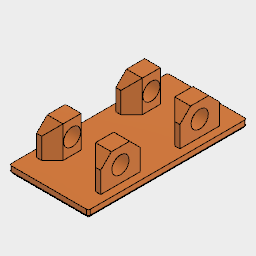
prusa_i3_bear_upgrade (Autodesk Fusion 360 archive; units mm, degrees)
design "end_cap"
Autodesk Fusion 360 part; units mm, degrees
sketch "base" plane through (0, 0, 0) normal (0, 0, 1) x (1, 0, 0)
  line L0 (0, 0) -> (20, 0)
  line L1 (20, 0) -> (20, 40)
  line L2 (20, 40) -> (0, 40)
  line L3 (0, 40) -> (0, 0)
  line L4 (10, 0) -> (10, 40) construction
  line L5 (1.9, 15) -> (5.9, 15)
  line L6 (5.9, 15) -> (5.9, 5)
  line L7 (5.9, 5) -> (1.9, 5)
  line L8 (1.9, 5) -> (1.9, 15)
  line L9 (14.1, 15) -> (18.1, 15)
  line L10 (18.1, 15) -> (18.1, 5)
  line L11 (18.1, 5) -> (14.1, 5)
  line L12 (14.1, 5) -> (14.1, 15)
  line L13 (0, 10) -> (20, 10) construction
  line L14 (0, 20) -> (20, 20) construction
  line L15 (5.9, 25) -> (5.9, 35)
  line L16 (5.9, 35) -> (1.9, 35)
  line L17 (1.9, 25) -> (5.9, 25)
  line L18 (1.9, 35) -> (1.9, 25)
  line L19 (18.1, 25) -> (18.1, 35)
  line L20 (18.1, 35) -> (14.1, 35)
  line L21 (14.1, 25) -> (18.1, 25)
  line L22 (14.1, 35) -> (14.1, 25)
  dimension "d2505" = 20
  dimension "d2506" = 40
  dimension "d2525" = 0
  dimension "d2526" = 0
  dimension "d2527" = 0
  dimension "d2528" = 0
  dimension "d2539" = 0
  dimension "d2540" = 0
  dimension "d2541" = 0
  dimension "d2542" = 0
  dimension "d2551" = 0
  dimension "d2552" = 0
  dimension "d2553" = 0
  dimension "d2554" = 0
  dimension "d2563" = 0
  dimension "d2564" = 0
  dimension "d2565" = 0
  dimension "d2566" = 0
  dimension "d2" = 10
  dimension "d3" = 4
  dimension "d4" = 10
  dimension "d5" = 4
  dimension "d6" = 10
  dimension "d7" = 1.9
  dimension "d8" = 1.9
  dimension "d12" = 20
  measures "d2505" distance of L0.start L0.end
  measures "d2506" distance of L0.start L2.end
  measures "d2" distance of L5.end L6.end
  measures "d3" distance of L5.start L5.end
  measures "d4" distance of L9.start L11.end
  measures "d5" distance of L9.start L9.end
  measures "d6" distance of L0 L13
  measures "d7" distance of L3 L8
  measures "d8" distance of L1 L10
  measures "d12" distance of L2 L14
extrude "Extrude1" add sketch "base" along normal blind 2 contours L0 L1 L2 L3 | L5 L6 L7 L8 | L9 L10 L11 L12 | L15 L16 L17 L18 | L19 L20 L21 L22
extrude "Extrude2" add sketch "base" along normal up to surface (10 mm away) contours L5 L6 L7 L8 | L9 L10 L11 L12 | L15 L16 L17 L18 | L19 L20 L21 L22
sketch "holes" plane through (0, 0, 0) normal (-1, 0, 0) x (0, -1, 0)
  line L0 (0, 2) -> (-40, 2)
  line L1 (-15, 2) -> (-15, 10)
  line L2 (-15, 2) -> (-5, 2)
  line L3 (-5, 2) -> (-5, 10)
  line L4 (-5, 10) -> (-15, 10)
  line L5 (-15, 10) -> (-15, 2)
  line L6 (-15, 6) -> (-5, 6) construction
  circle A0 centre (-10, 6) radius 2.175
  line L7 (-40, 0) -> (0, 0)
  line L8 (0, 0) -> (0, 2)
  line L9 (-40, 2) -> (-40, 0)
  line L10 (-35, 2) -> (-25, 2)
  line L11 (-25, 2) -> (-25, 10)
  line L12 (-25, 10) -> (-35, 10)
  line L13 (-35, 10) -> (-35, 2)
  line L14 (-35, 6) -> (-25, 6) construction
  circle A1 centre (-30, 6) radius 2.175
  dimension "d9" = 4.35
  dimension "d13" = 4.35
  measures "d9" diameter of A0
  measures "d13" diameter of A1
extrude "Extrude5" cut sketch "holes" against normal up to surface (20 mm away) contours A0 | A1
fillet "Fillet1" radius 0.5 4 edges at (20, 40, 1) (0, 40, 1) (0, 0, 1) (20, 0, 1)
chamfer "Chamfer1" distance 2.7 angle 45 16 edges at (5.9, 5, 6) (3.9, 5, 10) (3.9, 15, 10) (5.9, 15, 6) (16.1, 15, 10) (16.1, 5, 10) (14.1, 5, 6) (14.1, 15, 6) (5.9, 25, 6) (14.1, 25, 6) (3.9, 25, 10) (16.1, 25, 10) (16.1, 35, 10) (14.1, 35, 6) (5.9, 35, 6) (3.9, 35, 10)
sketch "bear" plane through (0, 0, 0) normal (0, 0, -1) x (1, 0, 0)
  arc A0 (20, -0.5) -> (19.5, 0) centre (19.5, -0.5) ccw
  line L0 (19.5, 0) -> (0.5, 0)
  arc A1 (0.5, 0) -> (0, -0.5) centre (0.5, -0.5) ccw
  line L1 (0, -0.5) -> (0, -39.5)
  arc A2 (0, -39.5) -> (0.5, -40) centre (0.5, -39.5) ccw
  line L2 (0.5, -40) -> (19.5, -40)
  arc A3 (19.5, -40) -> (20, -39.5) centre (19.5, -39.5) ccw
  line L3 (20, -39.5) -> (20, -0.5)
  spline S0 degree 5 poles (9.966, -9.8106) (10.0307, -9.8106) (10.1684, -9.8018) (10.4002, -9.7624) (10.7537, -9.6582) (11.2372, -9.4515) (11.7261, -9.1858) (12.1914, -8.8873) (12.6273, -8.5936) (13.0463, -8.3489) (13.4677, -8.1963) (13.9085, -8.1718) (14.3719, -8.2972) (14.8428, -8.5761) (15.2947, -8.999) (15.695, -9.5463) (16.0101, -10.1916) (16.2113, -10.9054) (16.2794, -11.6578) (16.209, -12.4202) (16.0114, -13.168) (15.7222, -13.8822) (15.3966, -14.5517) (15.1369, -15.1757) (15.0089, -15.7636) (15.0284, -16.33) (15.1825, -16.8916) (15.4362, -17.4636) (15.7454, -18.0556) (16.0669, -18.6687) (16.3609, -19.2975) (16.5931, -19.9328) (16.7373, -20.5637) (16.7772, -21.1803) (16.7099, -21.7758) (16.546, -22.3484) (16.3066, -22.8993) (16.0201, -23.4315) (15.7195, -23.9484) (15.4391, -24.4521) (15.2113, -24.9429) (15.0636, -25.4207) (15.0135, -25.887) (15.066, -26.3466) (15.2079, -26.8103) (15.4098, -27.293) (15.6325, -27.8087) (15.8324, -28.3659) (15.9677, -28.9632) (16.0042, -29.5842) (15.9174, -30.2003) (15.6941, -30.777) (15.3335, -31.2788) (14.8486, -31.674) (14.2686, -31.9409) (13.634, -32.0695) (12.9888, -32.0625) (12.3726, -31.9358) (11.8135, -31.7192) (11.319, -31.4585) (10.8754, -31.2111) (10.5431, -31.0686) (10.2967, -31.0125) (10.1323, -31) (10.05, -31) knots 0 0 0 0 0 0 0.01666667 0.03333333 0.05 0.06666667 0.08333333 0.1 0.11666667 0.13333333 0.15 0.16666667 0.18333333 0.2 0.21666667 0.23333333 0.25 0.26666667 0.28333333 0.3 0.31666667 0.33333333 0.35 0.36666667 0.38333333 0.4 0.41666667 0.43333333 0.45 0.46666667 0.48333333 0.5 0.51666667 0.53333333 0.55 0.56666667 0.58333333 0.6 0.61666667 0.63333333 0.65 0.66666667 0.68333333 0.7 0.71666667 0.73333333 0.75 0.76666667 0.78333333 0.8 0.81666667 0.83333333 0.85 0.86666667 0.88333333 0.9 0.91666667 0.93333333 0.95 0.96666667 0.98333333 1 1 1 1 1 1
  line L4 (8.166, -9.8106) -> (11.766, -9.8106)
  line L5 (16.65, -11.8) -> (14.3026, -16.9967)
  line L6 (12.25, -31) -> (7.85, -31)
  line L7 (9.966, -9.8106) -> (10.05, -31) construction
  spline S1 degree 5 poles (9.966, -9.8106) (9.9013, -9.8111) (9.7635, -9.8034) (9.5314, -9.7658) (9.1772, -9.6645) (8.692, -9.4616) (8.2011, -9.1997) (7.7334, -8.9049) (7.2952, -8.6148) (6.8742, -8.3734) (6.4517, -8.2241) (6.0107, -8.2032) (5.5482, -8.3322) (5.0796, -8.6148) (4.631, -9.0413) (4.2351, -9.5917) (3.9251, -10.2395) (3.7296, -10.9549) (3.6674, -11.7078) (3.7439, -12.4696) (3.9475, -13.2158) (4.2422, -13.9277) (4.5732, -14.5946) (4.8378, -15.2165) (4.9705, -15.8034) (4.9555, -16.3699) (4.8058, -16.9328) (4.5567, -17.5067) (4.2522, -18.1012) (3.9355, -18.7168) (3.6465, -19.3479) (3.4193, -19.985) (3.2802, -20.617) (3.2451, -21.2339) (3.3172, -21.8288) (3.4856, -22.4002) (3.7294, -22.9492) (4.0201, -23.4791) (4.3248, -23.9935) (4.6092, -24.4951) (4.8408, -24.984) (4.9923, -25.4606) (5.0461, -25.9265) (4.9973, -26.3865) (4.859, -26.8513) (4.661, -27.3356) (4.4424, -27.8531) (4.2469, -28.4118) (4.1163, -29.0102) (4.0848, -29.6314) (4.1764, -30.2468) (4.4043, -30.8218) (4.7689, -31.3207) (5.2569, -31.712) (5.839, -31.9743) (6.4746, -32.0979) (7.1197, -32.0858) (7.7349, -31.9542) (8.2923, -31.7332) (8.7847, -31.4685) (9.2263, -31.2176) (9.5575, -31.0725) (9.8034, -31.0144) (9.9677, -31.0007) (10.05, -31) knots 0 0 0 0 0 0 0.01666667 0.03333333 0.05 0.06666667 0.08333333 0.1 0.11666667 0.13333333 0.15 0.16666667 0.18333333 0.2 0.21666667 0.23333333 0.25 0.26666667 0.28333333 0.3 0.31666667 0.33333333 0.35 0.36666667 0.38333333 0.4 0.41666667 0.43333333 0.45 0.46666667 0.48333333 0.5 0.51666667 0.53333333 0.55 0.56666667 0.58333333 0.6 0.61666667 0.63333333 0.65 0.66666667 0.68333333 0.7 0.71666667 0.73333333 0.75 0.76666667 0.78333333 0.8 0.81666667 0.83333333 0.85 0.86666667 0.88333333 0.9 0.91666667 0.93333333 0.95 0.96666667 0.98333333 1 1 1 1 1 1
  line L8 (11.766, -9.7963) -> (8.1661, -9.8249)
  line L9 (3.298, -11.8529) -> (5.6865, -17.0308)
  line L10 (7.8501, -31.0174) -> (12.2499, -30.9826)
  circle A4 centre (12.5483, -27.3765) radius 0.7448
  ellipse E0 centre (10.0265, -25.0801) end of major axis (8.2046, -25.0873) minor radius 1.3284
  line L11 (11.8485, -25.0728) -> (8.2046, -25.0873)
  line L12 (10.0213, -23.7517) -> (10.0318, -26.4085)
  circle A5 centre (7.523, -27.3965) radius 0.7448
  ellipse E1 centre (14.4043, -20.6952) end of major axis (14.4043, -18.6032) minor radius 1.5739
  line L13 (14.4043, -22.7872) -> (14.4043, -18.6032)
  line L14 (15.9782, -20.6952) -> (12.8304, -20.6952)
  ellipse E2 centre (5.6142, -20.73) end of major axis (5.5976, -18.6381) minor radius 1.5739
  ellipse E3 centre (13.9043, -11.1952) end of major axis (13.9043, -9.1032) minor radius 1.5739
  ellipse E4 centre (6.0388, -11.2264) end of major axis (6.0223, -9.1344) minor radius 1.5739
  point P0 (13.75, -8.2)
  point P1 (15.85, -9.9)
  point P2 (15.4763, -14.3983)
  point P3 (15.4416, -17.4507)
  point P4 (16.75, -21)
  point P5 (15.75, -23.9)
  point P6 (15.05, -26.1)
  point P7 (15.85, -28.5)
  point P8 (15.15, -31.4)
  point P9 (12.05, -31.8)
  point P10 (11.85, -9.1)
  point P11 (8.0764, -9.115)
  point P12 (6.1694, -8.23)
  point P13 (4.0829, -9.9466)
  point P14 (4.4923, -14.4419)
  point P15 (4.5511, -17.4939)
  point P16 (3.2709, -21.0534)
  point P17 (4.2939, -23.9454)
  point P18 (5.0113, -26.1398)
  point P19 (4.2304, -28.5461)
  point P20 (4.9533, -31.4404)
  point P21 (8.0564, -31.8158)
extrude "Extrude4" cut sketch "bear" against normal blind 1 contours S0 S1
chamfer "Chamfer2" distance 0.7 angle 35 8 edges at (10, 40, 0) (0.1464, 39.8536, 0) (0, 20, 0) (0.1464, 0.1464, 0) (10, 0, 0) (19.8536, 0.1464, 0) (20, 20, 0) (19.8536, 39.8536, 0) measured on face at (13.1667, 40, 1.3333) measured on face at (0.0141, 39.6179, 0.6667) measured on face at (0, 26.5, 1.3333) measured on face at (0.4762, 0.0006, 0.6667) measured on face at (6.8333, 0, 0.6667) measured on face at (19.8619, 0.155, 0.6667) measured on face at (20, 13.5, 1.3333) measured on face at (19.991, 39.5946, 0.6667)
equation "d4 = d2"
equation "d5 = d3"
equation "d8 = d7"
equation "d13 = d9"

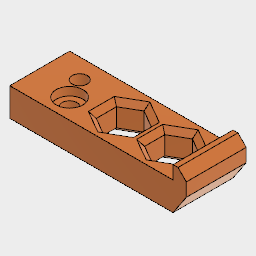
design "psu_upper_mount"
Autodesk Fusion 360 part; units mm, degrees
sketch "base" plane through (0, 0, 0) normal (0, 0, 1) x (1, 0, 0)
  circle A0 centre (9, 12.025) radius 2.25
  circle A1 centre (12, 5.975) radius 2.25
  circle A2 centre (12, 5.975) radius 4
  circle A3 centre (9, 12.025) radius 3.6 construction
  line L0 (5.8823, 10.225) -> (9, 8.425)
  line L1 (9, 8.425) -> (12.1177, 10.225)
  line L2 (12.1177, 10.225) -> (12.1177, 13.825)
  line L3 (12.1177, 13.825) -> (9, 15.625)
  line L4 (9, 15.625) -> (5.8823, 13.825)
  line L5 (5.8823, 13.825) -> (5.8823, 10.225)
  line L6 (0, 18) -> (53, 18)
  line L7 (53, 18) -> (53, 0)
  line L8 (53, 0) -> (0, 0)
  line L9 (0, 0) -> (0, 18)
  line L10 (49, 18) -> (49, 0)
  line L11 (0, 9) -> (49, 9) construction
  point P0 (9, 12.025)
  dimension "d1" = 4.5
  dimension "d2" = 4.5
  dimension "d3" = 8
  dimension "d6" = 7.2
  dimension "d8" = 4
  dimension "d9" = 18
  dimension "d22" = 49
  dimension "d23" = 40
  dimension "d31" = 6.05
  dimension "d33" = 3
  dimension "d34" = 3.025
  measures "d1" diameter of A0
  measures "d2" diameter of A1
  measures "d3" diameter of A2
  measures "d6" diameter of A3
  measures "d8" distance of L7 L10
  measures "d9" distance of L6.start L8.end
  measures "d22" distance of L9 L10
  measures "d23" distance of P0 L10
  measures "d31" distance of P0 A1.centre
  measures "d33" distance of P0 A1.centre
  measures "d34" distance of P0 L11.start
extrude "Extrude1" add sketch "base" along normal blind 8.5 contours A2 L0 L1 | A2 L0 L1 | A2 L0 L1 L2 L3 L4 L5 | L6 L8 L9 L10
extrude "Extrude2" add sketch "base" along normal up to surface (12.5 mm away) contours L6 L7 L8 L10
extrude "Extrude3" cut sketch "base" along normal blind 4 contours A2 L0 L1 | A2 L0 L1 L2 L3 L4 L5 picked at (10.5961, 9.4215)
extrude "Extrude4" cut sketch "base" against normal blind 2.5 from surface at 8.5 contours A2 L0 L1 | A2 L0 L1
sketch "poly" plane through (0, 0, 8.5) normal (0, 0, 1) x (-1, 0, 0)
  circle A0 centre (-12, -5.975) radius 4
  circle A1 centre (-9, -12.025) radius 2.25
  line L0 (-49, -18) -> (0, -18)
  line L1 (0, -18) -> (0, 0)
  line L2 (0, 0) -> (-49, 0)
  line L3 (-49, 0) -> (-49, -18)
  line L4 (-49, -18) -> (-49, 0)
  line L5 (-49, -9) -> (-16, -9) construction
  line L6 (-49, -18) -> (0, -18)
  line L7 (0, 0) -> (-49, 0)
  line L8 (-16, -18) -> (-16, 0) construction
  line L9 (-25.25, -15.0622) -> (-20, -12.0311)
  line L10 (-20, -12.0311) -> (-20, -5.9689)
  line L11 (-20, -5.9689) -> (-25.25, -2.9378)
  line L12 (-25.25, -2.9378) -> (-30.5, -5.9689)
  line L13 (-30.5, -5.9689) -> (-30.5, -12.0311)
  line L14 (-30.5, -12.0311) -> (-25.25, -15.0622)
  line L15 (-34.5, -12.0311) -> (-34.5, -5.9689)
  line L16 (-34.5, -5.9689) -> (-39.75, -2.9378)
  line L17 (-39.75, -2.9378) -> (-45, -5.9689)
  line L18 (-45, -5.9689) -> (-45, -12.0311)
  line L19 (-45, -12.0311) -> (-39.75, -15.0622)
  line L20 (-39.75, -15.0622) -> (-34.5, -12.0311)
  line L21 (-39.75, -9) -> (-42.375, -13.5466) construction
  circle A2 centre (-12, -5.975) radius 4
  point P0 (-25.25, -9)
  point P1 (-39.75, -9)
  dimension "d25" = 4
  dimension "d26" = 4
  dimension "d27" = 4
  measures "d25" distance of L8 L10
  measures "d26" distance of L3 L18
  measures "d27" distance of L13 L15
extrude "Extrude5" cut sketch "poly" against normal up to surface (8.5 mm away) contours L9 L10 L11 L12 L13 L14 | L15 L16 L17 L18 L19 L20
chamfer "Chamfer1" distance 2.5 angle 45 1 edges at (53, 9, 12.5)
chamfer "Chamfer2" distance 1.5 angle 45 24 edges at (27.875, 4.4534, 8.5) (30.5, 9, 8.5) (27.875, 13.5466, 8.5) (22.625, 13.5466, 8.5) (20, 9, 8.5) (22.625, 4.4534, 8.5) (22.625, 4.4534, 0) (27.875, 4.4534, 0) (30.5, 9, 0) (34.5, 9, 8.5) (37.125, 4.4534, 0) (37.125, 4.4534, 8.5) (42.375, 4.4534, 0) (42.375, 4.4534, 8.5) (45, 9, 0) (45, 9, 8.5) (42.375, 13.5466, 8.5) (37.125, 13.5466, 8.5) (27.875, 13.5466, 0) (22.625, 13.5466, 0) (20, 9, 0) (37.125, 13.5466, 0) (34.5, 9, 0) (42.375, 13.5466, 0) measured on face at (2.2833, 9.7873, 8.5) measured on face at (2.2833, 9.7873, 8.5) measured on face at (2.2833, 9.7873, 8.5) measured on face at (2.2833, 9.7873, 8.5) measured on face at (2.2833, 9.7873, 8.5) measured on face at (2.2833, 9.7873, 8.5) measured on face at (50.3333, 10.0104, 0) measured on face at (50.3333, 10.0104, 0) measured on face at (50.3333, 10.0104, 0) measured on face at (2.2833, 9.7873, 8.5) measured on face at (50.3333, 10.0104, 0) measured on face at (2.2833, 9.7873, 8.5) measured on face at (50.3333, 10.0104, 0) measured on face at (2.2833, 9.7873, 8.5) measured on face at (50.3333, 10.0104, 0) measured on face at (2.2833, 9.7873, 8.5) measured on face at (2.2833, 9.7873, 8.5) measured on face at (2.2833, 9.7873, 8.5) measured on face at (50.3333, 10.0104, 0) measured on face at (50.3333, 10.0104, 0) measured on face at (50.3333, 10.0104, 0) measured on face at (50.3333, 10.0104, 0) measured on face at (50.3333, 10.0104, 0) measured on face at (50.3333, 10.0104, 0)
chamfer "Chamfer3" distance 4 distance2 6 1 edges at (53, 9, 0) measured on face at (50.8333, 7.701, 0)
ref_plane "WorkPlane1" through (26.5, 9, 4.25) normal (0, 0, -1) x (-1, 0, 0)
sketch "waste_pocket" plane through (24.5, 9, 4.25) normal (0, 0, -1) x (1, 0, 0)
  circle A0 centre (-12.5, 3.025) radius 4
  line L0 (-12.3823, -4.825) -> (-15.5, -6.625)
  line L1 (-12.3823, -1.225) -> (-12.3823, -4.825)
  line L2 (-15.5, 0.575) -> (-12.3823, -1.225)
  line L3 (-18.6177, -1.225) -> (-15.5, 0.575)
  line L4 (-18.6177, -4.825) -> (-18.6177, -1.225)
  line L5 (-15.5, -6.625) -> (-18.6177, -4.825)
  line L6 (-6, 3.8971) -> (-6, -3.8971)
  line L7 (-6, -3.8971) -> (0.75, -7.7942)
  line L8 (0.75, 7.7942) -> (-6, 3.8971)
  line L9 (-23, -7) -> (-21.6177, -7)
  line L10 (-18.5, 7) -> (-23, 7)
  line L11 (-23, 7) -> (-23, -7)
  line L12 (-24.5, -9) -> (-24.5, 9)
  line L13 (-24.5, 9) -> (24.5, 9)
  line L14 (24.5, -9) -> (-24.5, -9)
  line L15 (-9.3823, -7) -> (-7.5, -7)
  line L16 (-7.5, -7) -> (-7.5, -2.1014)
  line L17 (-7.5, -2.1014) -> (-9.3823, -2.1014)
  line L18 (-9.3823, -2.1014) -> (-9.3823, -7)
  line L19 (7.5, -3.8971) -> (0.75, -7.7942)
  line L20 (15.25, -7.7942) -> (8.5, -3.8971)
  line L21 (0.75, 7.7942) -> (7.5, 3.8971)
  line L22 (8.5, 3.8971) -> (15.25, 7.7942)
  line L23 (22, -3.8971) -> (15.25, -7.7942)
  line L24 (15.25, 7.7942) -> (22, 3.8971)
  line L25 (24.5, 9) -> (24.5, -9)
  line L26 (5.1256, -7) -> (8, -5.3405)
  line L27 (8, -5.3405) -> (10.8744, -7)
  line L28 (10.8744, -7) -> (5.1256, -7)
  line L29 (5.1256, 7) -> (8, 5.3405)
  line L30 (8, 5.3405) -> (10.8744, 7)
  line L31 (10.8744, 7) -> (5.1256, 7)
  line L32 (19.6256, 7) -> (22.5, 5.3405)
  line L33 (22.5, 5.3405) -> (22.5, 7)
  line L34 (22.5, 7) -> (19.6256, 7)
  line L35 (19.6256, -7) -> (22.5, -5.3405)
  line L36 (22.5, -5.3405) -> (22.5, -7)
  line L37 (22.5, -7) -> (19.6256, -7)
  line L38 (-21.6177, -7) -> (-21.6177, 0.5071)
  line L39 (-21.6177, 0.5071) -> (-18.5, 2.3071)
  line L40 (-18.5, 2.3071) -> (-18.5, 7)
  dimension "d41" = 1.5
  dimension "d42" = 2
  dimension "d43" = 2
  dimension "d47" = 1.5
  dimension "d48" = 3
  dimension "d49" = 2
  dimension "d52" = 1.5
  dimension "d53" = 1.5
  dimension "d54" = 1.5
  dimension "d55" = 1.5
  dimension "d56" = 1.5
  dimension "d57" = 1.5
  dimension "d58" = 2
  dimension "d59" = 2
  dimension "d60" = 3
  dimension "d61" = 3
  dimension "d62" = 2
  measures "d41" distance of L11 L12
  measures "d42" distance of L10 L13
  measures "d43" distance of L9 L14
  measures "d47" distance of L6 L16
  measures "d48" distance of L0.start L18
  measures "d49" distance of A0 L17.end
  measures "d52" distance of L21 L29
  measures "d53" distance of L22 L30
  measures "d54" distance of L24 L32
  measures "d55" distance of L19 L26
  measures "d56" distance of L20 L27
  measures "d57" distance of L23 L35
  measures "d58" distance of L25 L36
  measures "d59" distance of L25 L33
  measures "d60" distance of L3 L39
  measures "d61" distance of L4 L38
  measures "d62" distance of A0 L40
extrude "Extrude6" cut sketch "waste_pocket" along normal mid plane 4.5 contours L9 L10 L11 L38 L39 L40 | L15 L16 L17 L18 | L26 L27 L28 | L29 L30 L31 | L32 L33 L34 | L35 L36 L37
equation "d13 = thickness"
equation "d23 = 55 mm - 15 mm"
equation "d26 = d25"
equation "d34 = d31 / 2"
equation "thickness = 8.5 mm"
equation "d50 = thickness - ( 2 * 2 ) * 1 mm"
equation "d53 = d52"
equation "d54 = d52"
equation "d55 = d52"
equation "d56 = d52"
equation "d57 = d52"
